Support CI (Autodesk Fusion 360 design; units mm, degrees)
Autodesk Fusion 360 part; units mm, degrees
sketch "Sketch1" plane through (0, 0, 0) normal (0, 0, 1) x (1, 0, 0)
  line L0 (32.5, -45) -> (-32.5, -45)
  line L1 (-36, -41.5) -> (-36, 41.5)
  line L2 (-32.5, 45) -> (32.5, 45)
  line L3 (36, 41.5) -> (36, -41.5)
  line L4 (36, -45) -> (-36, 45) construction
  line L5 (-36, -45) -> (36, 45) construction
  line L6 (32.5, -41.5) -> (-32.5, -41.5) construction
  line L7 (-32.5, -41.5) -> (-32.5, 41.5) construction
  line L8 (-32.5, 41.5) -> (32.5, 41.5) construction
  line L9 (32.5, 41.5) -> (32.5, -41.5) construction
  line L10 (32.5, -41.5) -> (-32.5, 41.5) construction
  line L11 (-32.5, -41.5) -> (32.5, 41.5) construction
  circle A0 centre (-32.5, 41.5) radius 3.5
  circle A1 centre (32.5, 41.5) radius 3.5
  circle A2 centre (-32.5, -41.5) radius 3.5
  circle A3 centre (32.5, -41.5) radius 3.5
  circle A4 centre (-32.5, 41.5) radius 1.6
  circle A5 centre (32.5, 41.5) radius 1.6
  circle A6 centre (32.5, -41.5) radius 1.6
  circle A7 centre (-32.5, -41.5) radius 1.6
  arc A8 (-32.5, 45) -> (-36, 41.5) centre (-32.5, 41.5) ccw
  arc A9 (36, 41.5) -> (32.5, 45) centre (32.5, 41.5) ccw
  arc A10 (32.5, -45) -> (36, -41.5) centre (32.5, -41.5) ccw
  arc A11 (-36, -41.5) -> (-32.5, -45) centre (-32.5, -41.5) ccw
  line L12 (30, -27.5) -> (-30, -27.5) construction
  line L13 (-30, -27.5) -> (-30, 27.5) construction
  line L14 (-30, 27.5) -> (30, 27.5) construction
  line L15 (30, 27.5) -> (30, -27.5) construction
  line L16 (30, -27.5) -> (-30, 27.5) construction
  line L17 (-30, -27.5) -> (30, 27.5) construction
  circle A12 centre (-30, 27.5) radius 1.6
  circle A13 centre (0, 27.5) radius 1.6
  circle A14 centre (30, 27.5) radius 1.6
  circle A15 centre (-30, -27.5) radius 1.6
  circle A16 centre (0, -27.5) radius 1.6
  circle A17 centre (30, -27.5) radius 1.6
  line L18 (-1.5, 35) -> (-1.5, -35)
  arc A18 (-1.5, -35) -> (1.5, -35) centre (0, -35) ccw
  line L19 (1.5, -35) -> (1.5, 35)
  arc A19 (1.5, 35) -> (-1.5, 35) centre (0, 35) ccw
  line L20 (0, 35) -> (0, -35) construction
  line L21 (-24.5, 35) -> (-24.5, -35)
  arc A20 (-24.5, -35) -> (-21.5, -35) centre (-23, -35) ccw
  line L22 (-21.5, -35) -> (-21.5, 35)
  arc A21 (-21.5, 35) -> (-24.5, 35) centre (-23, 35) ccw
  line L23 (-16.8333, 35) -> (-16.8333, -35)
  arc A22 (-16.8333, -35) -> (-13.8333, -35) centre (-15.3333, -35) ccw
  line L24 (-13.8333, -35) -> (-13.8333, 35)
  arc A23 (-13.8333, 35) -> (-16.8333, 35) centre (-15.3333, 35) ccw
  line L25 (-9.1667, 35) -> (-9.1667, -35)
  arc A24 (-9.1667, -35) -> (-6.1667, -35) centre (-7.6667, -35) ccw
  line L26 (-6.1667, -35) -> (-6.1667, 35)
  arc A25 (-6.1667, 35) -> (-9.1667, 35) centre (-7.6667, 35) ccw
  line L27 (6.1667, 35) -> (6.1667, -35)
  arc A26 (6.1667, -35) -> (9.1667, -35) centre (7.6667, -35) ccw
  line L28 (9.1667, -35) -> (9.1667, 35)
  arc A27 (9.1667, 35) -> (6.1667, 35) centre (7.6667, 35) ccw
  line L29 (13.8333, 35) -> (13.8333, -35)
  arc A28 (13.8333, -35) -> (16.8333, -35) centre (15.3333, -35) ccw
  line L30 (16.8333, -35) -> (16.8333, 35)
  arc A29 (16.8333, 35) -> (13.8333, 35) centre (15.3333, 35) ccw
  line L31 (21.5, 35) -> (21.5, -35)
  arc A30 (21.5, -35) -> (24.5, -35) centre (23, -35) ccw
  line L32 (24.5, -35) -> (24.5, 35)
  arc A31 (24.5, 35) -> (21.5, 35) centre (23, 35) ccw
  dimension "d1" = 72
  dimension "d2" = 90
  dimension "d3" = 65
  dimension "d4" = 83
  dimension "d5" = 7
  dimension "d6" = 7
  dimension "d7" = 7
  dimension "d8" = 7
  dimension "d9" = 3.2
  dimension "d10" = 3.2
  dimension "d11" = 3.2
  dimension "d12" = 3.2
  dimension "d13" = 3.5
  dimension "d14" = 60
  dimension "d15" = 55
  dimension "d16" = 3.2
  dimension "d17" = 3.2
  dimension "d18" = 3.2
  dimension "d19" = 3.2
  dimension "d20" = 3.2
  dimension "d21" = 3.2
  dimension "d22" = 3
  dimension "d25" = 23
  dimension "d26" = 0
  dimension "d27" = 70
  constraint horizontal L0
  constraint perpendicular L0 L1
  constraint parallel L0 L2
  constraint parallel L1 L3
  constraint coincident L4 origin
  constraint coincident L5 origin
  constraint horizontal L6
  constraint perpendicular L6 L7
  constraint parallel L6 L8
  constraint parallel L7 L9
  constraint coincident L10 origin
  constraint coincident L11 origin
  constraint coincident L7.end L8.start
  constraint coincident L8.end L9.start
  constraint coincident L6.end L7.start
  constraint coincident L6.start L9.end
  constraint concentric A0 A4
  constraint concentric A3 A6
  constraint concentric A2 A7
  constraint coincident L4.end L2
  constraint coincident L4.end L1
  constraint tangent L2 A8
  constraint tangent L1 A8
  constraint coincident L5.end L2
  constraint coincident L5.end L3
  constraint tangent L2 A9
  constraint tangent L3 A9
  constraint equal A8 A9
  constraint coincident L4.start L3
  constraint coincident L4.start L0
  constraint tangent L3 A10
  constraint tangent L0 A10
  constraint equal A8 A10
  constraint coincident L5.start L0
  constraint coincident L5.start L1
  constraint tangent L0 A11
  constraint tangent L1 A11
  constraint equal A8 A11
  constraint horizontal L12
  constraint perpendicular L12 L13
  constraint parallel L12 L14
  constraint parallel L13 L15
  constraint coincident L16 origin
  constraint coincident L17 origin
  constraint coincident L13.end L14.start
  constraint midpoint L14 A13.centre
  constraint coincident L14.end L15.start
  constraint coincident L12.end L13.start
  constraint midpoint L12 A16.centre
  constraint coincident L12.start L15.end
  constraint tangent L18 A18
  constraint tangent A18 L19
  constraint parallel L18 L19
  constraint tangent L19 A19
  constraint tangent L18 A19
  constraint vertical L20
  constraint midpoint L20 origin
  measures "d1" distance of L4.end L5.end
  measures "d2" distance of L5.start L4.end
  measures "d3" distance of L7.end L8.end
  measures "d4" distance of L6.end L7.end
  measures "d5" diameter of A0
  measures "d6" diameter of A1
  measures "d7" diameter of A2
  measures "d8" diameter of A3
  measures "d9" diameter of A4
  measures "d10" diameter of A5
  measures "d11" diameter of A6
  measures "d12" diameter of A7
  measures "d13" radius of A8
  measures "d14" distance of L13.end L14.end
  measures "d15" distance of L12.end L13.end
  measures "d16" diameter of A12
  measures "d17" diameter of A13
  measures "d18" diameter of A14
  measures "d19" diameter of A15
  measures "d20" diameter of A16
  measures "d21" diameter of A17
  measures "d22" diameter of A18
  measures "d27" distance of A19.centre A18.centre
extrude "Extrude1" add sketch "Sketch1" against normal blind 3 contours L0 L1 L2 L3 A0 A1 A2 A3 | A3 A10 | A2 A11 | A1 A9 | A0 A8 | A13 L18 L19 A19 | A13 A16 L18 L19 | A16 L18 A18 L19
extrude "Extrude2" add sketch "Sketch1" along normal blind 10 contours A3 A10 | A2 A11 | A1 A9 | A0 A8
fillet "Fillet1" radius 4 4 edges at (-30.0251, -39.0251, 0) (-30.0251, 39.0251, 0) (30.0251, 39.0251, 0) (30.0251, -39.0251, 0)
